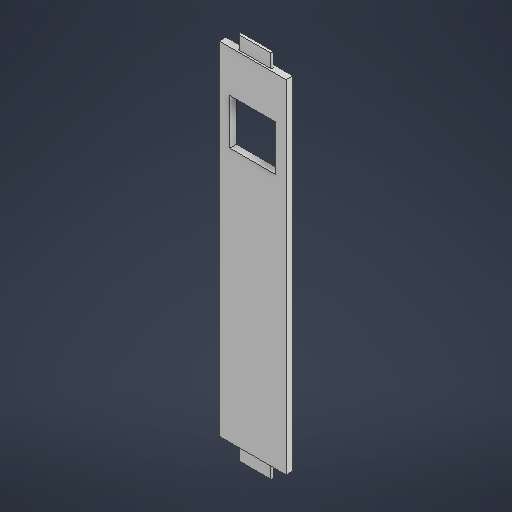
# Autodesk Inventor part: partttt
Saved by Autodesk Inventor 2026.2 (Build 302298010, 298A)
## iProperties
Created: 2026-03-03
Part Number: partttt
Material: Generic
Document SubType Name: Modeling
Designer: shahd
Density: 1 g/cm^3
Appearance: Default
Author: shahd
Autodesk Inventor part; units mm, degrees
ref_plane "YZ Plane" through (0, 0, 0) normal (1, 0, 0) x (0, 1, 0)
ref_plane "XZ Plane" through (0, 0, 0) normal (0, 1, 0) x (-1, 0, 0)
ref_plane "XY Plane" through (0, 0, 0) normal (0, 0, 1) x (1, 0, 0)
sketch "Sketch1" plane through (0, 0, 0) normal (0, 0, 1) x (1, 0, 0)
  line L0 (0, 0) -> (50, 0)
  line L1 (50, 0) -> (50, 255.203)
  line L2 (50, 255.203) -> (0, 255.203)
  line L3 (0, 255.203) -> (0, 0)
  line L4 (8, 224) -> (42, 224)
  line L5 (42, 224) -> (42, 190)
  line L6 (42, 190) -> (8, 190)
  line L7 (8, 190) -> (8, 224)
  point P0 (25, 255.203)
  dimension "d0" = 50
  dimension "d1" = 255.203
  dimension "d8" = 34
  dimension "d9" = 34
  dimension "d10" = 8
  dimension "d12" = 190
  constraints: 16 end point, 4 parallel, 2 horizontal, 2 perpendicular, 1 coincident, 1 midpoint
  measures "d0" distance of L2.end L1.end
  measures "d1" distance of L1.end L0.end
  measures "d8" distance of L4.start L4.end
  measures "d9" distance of L6.end L4.start
  measures "d10" distance between parallel lines of L3 L7
  measures "d12" distance between parallel lines of L0 L6
extrude "Extrusion1" add sketch "Sketch1" along normal blind 5
sketch "Sketch2" plane through (0, 0, 0) normal (0, -1, 0) x (1, 0, 0)
  line L0 (13.5, 2.5) -> (36.5, 2.5) construction
  line L1 (13.5, 1.5) -> (36.5, 1.5)
  line L2 (36.5, 3.5) -> (13.5, 3.5)
  arc A0 (13.5, 3.5) -> (13.5, 1.5) centre (13.5, 2.5) ccw
  arc A1 (36.5, 1.5) -> (36.5, 3.5) centre (36.5, 2.5) ccw
  line L3 (0, 5) -> (50, 5) projected
  point P0 (0, 0)
  point P1 (25, 2.5)
  point P2 (37.5, 2.5)
  point P3 (12.5, 2.5)
  dimension "d13" = 2
  dimension "d21" = 25
  dimension "d22" = 25
  dimension "d23" = 2.5
  constraints: 8 end point, 6 point on circle, 4 tangent, 2 centre point, 1 horizontal, 1 midpoint, 1 parallel
  measures "d13" diameter of A1
  measures "d21" horizontal distance of point (0, 0) point (25, 2.5)
  measures "d22" distance of point (37.5, 2.5) point (12.5, 2.5)
  measures "d23" vertical distance of point (0, 0) point (25, 2.5)
extrude "Extrusion2" add sketch "Sketch2" along normal blind 10
sketch "Sketch4" plane through (0, 255.203, 0) normal (0, 1, 0) x (1, 0, 0)
  line L0 (36.5, -2.5) -> (13.5, -2.5) construction
  line L1 (36.5, -1.5) -> (13.5, -1.5)
  line L2 (13.5, -3.5) -> (36.5, -3.5)
  arc A0 (36.5, -3.5) -> (36.5, -1.5) centre (36.5, -2.5) ccw
  arc A1 (13.5, -1.5) -> (13.5, -3.5) centre (13.5, -2.5) ccw
  point P0 (0, 0)
  point P1 (25, -2.5)
  point P2 (12.5, -2.5)
  point P3 (37.5, -2.5)
  dimension "d24" = 2
  dimension "d26" = 25
  dimension "d28" = 2.5
  dimension "d29" = 25
  constraints: 8 end point, 6 point on circle, 4 tangent, 2 centre point, 1 horizontal, 1 midpoint, 1 parallel
  measures "d24" diameter of A1
  measures "d26" distance of point (12.5, -2.5) point (37.5, -2.5)
  measures "d28" vertical distance of point (25, -2.5) point (0, 0)
  measures "d29" horizontal distance of point (0, 0) point (25, -2.5)
extrude "Extrusion3" add sketch "Sketch4" along normal blind 10
body "Solid1"
